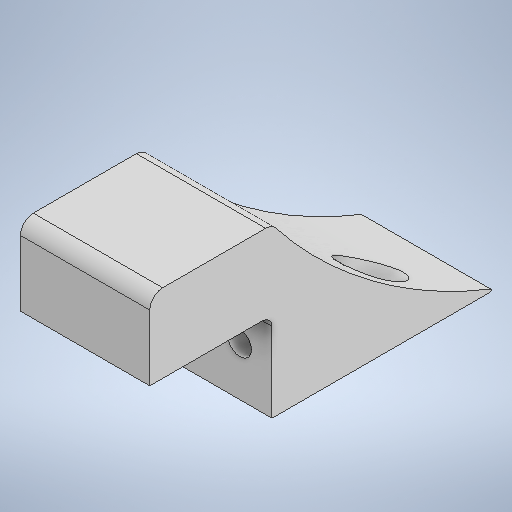
# Autodesk Inventor part: intake ramp piece
Saved by Autodesk Inventor 2025.2 (Build 292293000, 293)
## iProperties
Created: 2024-12-04
Part Number: intake ramp piece
Material: Generic
Document SubType Name: Modeling
Designer: Hunter Mathis
Density: 1 g/cm^3
Appearance: Default
Author: Hunter Mathis
## iProperties of the stored document Round intake ramp piece_3DPrint.ipt
Created: 2024-12-08
Part Number: Round intake ramp piece_3DPrint
Material: Generic
Document SubType Name: Modeling
Designer: AtuStem
Density: 1 g/cm^3
Appearance: Default
Author: AtuStem
Autodesk Inventor part; units mm, degrees
ref_plane "YZ Plane" through (0, 0, 0) normal (1, 0, 0) x (0, 1, 0)
ref_plane "XZ Plane" through (0, 0, 0) normal (0, 1, 0) x (-1, 0, 0)
ref_plane "XY Plane" through (0, 0, 0) normal (0, 0, 1) x (1, 0, 0)
sketch "Sketch24" plane through (0, 0, 0) normal (0, 0, 1) x (1, 0, 0)
  line L0 (0, 0) -> (177.8, 0)
  line L1 (177.8, 0) -> (177.8, 33.0962)
  line L2 (177.8, 33.0962) -> (0, 33.0962)
  line L3 (0, 33.0962) -> (0, 0)
  line L4 (88.9, 33.0962) -> (88.9, 0)
  line L5 (88.9, 0) -> (88.9, 7.3914)
  line L6 (88.9, 7.3914) -> (95.25, 7.3914)
  line L7 (94.488, 11.9634) -> (96.012, 11.9634)
  line L8 (97.536, 10.4394) -> (97.536, 8.9154)
  line L9 (96.012, 7.3914) -> (94.488, 7.3914)
  line L10 (92.964, 8.9154) -> (92.964, 10.4394)
  arc A0 (94.488, 11.9634) -> (92.964, 10.4394) centre (94.488, 10.4394) ccw
  arc A1 (97.536, 10.4394) -> (96.012, 11.9634) centre (96.012, 10.4394) ccw
  arc A2 (96.012, 7.3914) -> (97.536, 8.9154) centre (96.012, 8.9154) ccw
  arc A3 (92.964, 8.9154) -> (94.488, 7.3914) centre (94.488, 8.9154) ccw
  arc A4 (110.236, 10.4394) -> (108.712, 11.9634) centre (108.712, 10.4394) ccw
  arc A5 (108.712, 7.3914) -> (110.236, 8.9154) centre (108.712, 8.9154) ccw
  line L11 (108.712, 7.3914) -> (107.188, 7.3914)
  line L12 (105.664, 8.9154) -> (105.664, 10.4394)
  arc A6 (107.188, 11.9634) -> (105.664, 10.4394) centre (107.188, 10.4394) ccw
  arc A7 (105.664, 8.9154) -> (107.188, 7.3914) centre (107.188, 8.9154) ccw
  line L13 (107.188, 11.9634) -> (108.712, 11.9634)
  line L14 (110.236, 10.4394) -> (110.236, 8.9154)
  arc A8 (84.836, 10.4394) -> (83.312, 11.9634) centre (83.312, 10.4394) ccw
  arc A9 (83.312, 7.3914) -> (84.836, 8.9154) centre (83.312, 8.9154) ccw
  line L15 (83.312, 7.3914) -> (81.788, 7.3914)
  line L16 (80.264, 8.9154) -> (80.264, 10.4394)
  arc A10 (81.788, 11.9634) -> (80.264, 10.4394) centre (81.788, 10.4394) ccw
  arc A11 (80.264, 8.9154) -> (81.788, 7.3914) centre (81.788, 8.9154) ccw
  line L17 (81.788, 11.9634) -> (83.312, 11.9634)
  line L18 (84.836, 10.4394) -> (84.836, 8.9154)
  arc A12 (122.936, 10.4394) -> (121.412, 11.9634) centre (121.412, 10.4394) ccw
  arc A13 (121.412, 7.3914) -> (122.936, 8.9154) centre (121.412, 8.9154) ccw
  line L19 (121.412, 7.3914) -> (119.888, 7.3914)
  line L20 (118.364, 8.9154) -> (118.364, 10.4394)
  arc A14 (119.888, 11.9634) -> (118.364, 10.4394) centre (119.888, 10.4394) ccw
  arc A15 (118.364, 8.9154) -> (119.888, 7.3914) centre (119.888, 8.9154) ccw
  line L21 (119.888, 11.9634) -> (121.412, 11.9634)
  line L22 (122.936, 10.4394) -> (122.936, 8.9154)
  arc A16 (72.136, 10.4394) -> (70.612, 11.9634) centre (70.612, 10.4394) ccw
  arc A17 (70.612, 7.3914) -> (72.136, 8.9154) centre (70.612, 8.9154) ccw
  line L23 (70.612, 7.3914) -> (69.088, 7.3914)
  line L24 (67.564, 8.9154) -> (67.564, 10.4394)
  arc A18 (69.088, 11.9634) -> (67.564, 10.4394) centre (69.088, 10.4394) ccw
  arc A19 (67.564, 8.9154) -> (69.088, 7.3914) centre (69.088, 8.9154) ccw
  line L25 (69.088, 11.9634) -> (70.612, 11.9634)
  line L26 (72.136, 10.4394) -> (72.136, 8.9154)
  arc A20 (135.636, 10.4394) -> (134.112, 11.9634) centre (134.112, 10.4394) ccw
  arc A21 (134.112, 7.3914) -> (135.636, 8.9154) centre (134.112, 8.9154) ccw
  line L27 (134.112, 7.3914) -> (132.588, 7.3914)
  line L28 (131.064, 8.9154) -> (131.064, 10.4394)
  arc A22 (132.588, 11.9634) -> (131.064, 10.4394) centre (132.588, 10.4394) ccw
  arc A23 (131.064, 8.9154) -> (132.588, 7.3914) centre (132.588, 8.9154) ccw
  line L29 (132.588, 11.9634) -> (134.112, 11.9634)
  line L30 (135.636, 10.4394) -> (135.636, 8.9154)
  arc A24 (59.436, 10.4394) -> (57.912, 11.9634) centre (57.912, 10.4394) ccw
  arc A25 (57.912, 7.3914) -> (59.436, 8.9154) centre (57.912, 8.9154) ccw
  line L31 (57.912, 7.3914) -> (56.388, 7.3914)
  line L32 (54.864, 8.9154) -> (54.864, 10.4394)
  arc A26 (56.388, 11.9634) -> (54.864, 10.4394) centre (56.388, 10.4394) ccw
  arc A27 (54.864, 8.9154) -> (56.388, 7.3914) centre (56.388, 8.9154) ccw
  line L33 (56.388, 11.9634) -> (57.912, 11.9634)
  line L34 (59.436, 10.4394) -> (59.436, 8.9154)
  arc A28 (148.336, 10.4394) -> (146.812, 11.9634) centre (146.812, 10.4394) ccw
  arc A29 (146.812, 7.3914) -> (148.336, 8.9154) centre (146.812, 8.9154) ccw
  line L35 (146.812, 7.3914) -> (145.288, 7.3914)
  line L36 (143.764, 8.9154) -> (143.764, 10.4394)
  arc A30 (145.288, 11.9634) -> (143.764, 10.4394) centre (145.288, 10.4394) ccw
  arc A31 (143.764, 8.9154) -> (145.288, 7.3914) centre (145.288, 8.9154) ccw
  line L37 (145.288, 11.9634) -> (146.812, 11.9634)
  line L38 (148.336, 10.4394) -> (148.336, 8.9154)
  arc A32 (46.736, 10.4394) -> (45.212, 11.9634) centre (45.212, 10.4394) ccw
  arc A33 (45.212, 7.3914) -> (46.736, 8.9154) centre (45.212, 8.9154) ccw
  line L39 (45.212, 7.3914) -> (43.688, 7.3914)
  line L40 (42.164, 8.9154) -> (42.164, 10.4394)
  arc A34 (43.688, 11.9634) -> (42.164, 10.4394) centre (43.688, 10.4394) ccw
  arc A35 (42.164, 8.9154) -> (43.688, 7.3914) centre (43.688, 8.9154) ccw
  line L41 (43.688, 11.9634) -> (45.212, 11.9634)
  line L42 (46.736, 10.4394) -> (46.736, 8.9154)
  arc A36 (161.036, 10.4394) -> (159.512, 11.9634) centre (159.512, 10.4394) ccw
  arc A37 (159.512, 7.3914) -> (161.036, 8.9154) centre (159.512, 8.9154) ccw
  line L43 (159.512, 7.3914) -> (157.988, 7.3914)
  line L44 (156.464, 8.9154) -> (156.464, 10.4394)
  arc A38 (157.988, 11.9634) -> (156.464, 10.4394) centre (157.988, 10.4394) ccw
  arc A39 (156.464, 8.9154) -> (157.988, 7.3914) centre (157.988, 8.9154) ccw
  line L45 (157.988, 11.9634) -> (159.512, 11.9634)
  line L46 (161.036, 10.4394) -> (161.036, 8.9154)
  point P0 (95.25, 9.6774)
  point P1 (95.25, 7.3914)
  point P2 (107.95, 7.3914)
  point P3 (107.95, 9.6774)
  point P4 (107.95, 7.3914)
  point P5 (82.55, 7.3914)
  point P6 (82.55, 9.6774)
  point P7 (82.55, 7.3914)
  point P8 (120.65, 7.3914)
  point P9 (120.65, 9.6774)
  point P10 (120.65, 7.3914)
  point P11 (69.85, 7.3914)
  point P12 (69.85, 9.6774)
  point P13 (69.85, 7.3914)
  point P14 (133.35, 7.3914)
  point P15 (133.35, 9.6774)
  point P16 (133.35, 7.3914)
  point P17 (57.15, 7.3914)
  point P18 (57.15, 9.6774)
  point P19 (57.15, 7.3914)
  point P20 (146.05, 7.3914)
  point P21 (146.05, 9.6774)
  point P22 (146.05, 7.3914)
  point P23 (44.45, 7.3914)
  point P24 (44.45, 9.6774)
  point P25 (44.45, 7.3914)
  point P26 (158.75, 7.3914)
  point P27 (158.75, 9.6774)
  point P28 (158.75, 7.3914)
  dimension "d106" = 177.8
  dimension "d107" = 33.0962
  dimension "d119" = 7.3914
  dimension "d120" = 6.35
  dimension "d121" = 1.524
  dimension "d180" = 12.7
  constraints: 94 end point, 80 point on circle, 40 centre point, 8 tangent, 4 parallel, 3 equal radius, 3 horizontal, 3 midpoint, 3 perpendicular, 1 point on line, 207 other
  measures "d106" distance of L2.end L1.end
  measures "d107" distance of L0.end L1.end
  measures "d119" distance of L4.end L5.end
  measures "d120" distance of L5.end L6.end
  measures "d121" radius of A0
  measures "d180" distance of A1.centre A4.centre
sketch "Sketch26" plane through (0, 0, 0) normal (1, 0, 0) x (0, 1, 0)
  line L0 (0, 0) -> (0, -44.45)
  line L1 (33.0962, 0) -> (0, 0) projected
  arc A0 (33.0962, 0) -> (0, -44.45) centre (95.48, -80.9954) ccw
  dimension "d108" = 44.45
  dimension "d109" = 102.235
  constraints: 2 end point, 2 point on circle, 1 centre point, 1 vertical
  measures "d108" distance of L0.start L0.end
  measures "d109" radius of A0
extrude "Extrusion23" add sketch "Sketch26" along normal blind 177.8
sketch "Sketch27" plane through (0, 0, 0) normal (0, 0, 1) x (1, 0, 0)
  line L0 (0, 0) -> (44.45, 0)
  line L1 (0, 0) -> (177.8, 0) projected
  line L2 (44.45, 0) -> (44.45, 33.0962)
  line L3 (0, 33.0962) -> (177.8, 33.0962) projected
  arc A0 (0, 0) -> (44.45, 33.0962) centre (-36.5454, 95.48) ccw
  line L4 (0, 33.0962) -> (0, 0) projected
  line L5 (0, 0) -> (0, 33.0962)
  line L6 (0, 33.0962) -> (44.45, 33.0962)
  line L7 (0, 33.0962) -> (-19.05, 33.0962)
  line L8 (-19.05, 33.0962) -> (-19.05, 0)
  line L9 (-19.05, 0) -> (0, 0)
  line L10 (0, 0) -> (0, 33.0962)
  dimension "d112" = 44.45
  dimension "d113" = 102.235
  dimension "d114" = 19.05
  constraints: 16 end point, 3 equal length, 3 perpendicular, 2 point on circle, 2 point on line, 1 centre point, 1 horizontal
  measures "d112" distance of L0.start L0.end
  measures "d113" radius of A0
  measures "d114" distance of L9.end L8.end
revolve "Revolution1" [suppressed]
ref_plane "Work Plane3" through (88.9, 33.0962, 0) normal (-1, 0, 0) x (0, -1, 0)
mirror "Mirror1" [suppressed]
extrude "Extrusion24" add sketch "Sketch24" along normal blind 1.6002 contours A3 L10 A0 L7 A1 L8 A2 L9 L6 | L18 A9 L15 A11 L16 A10 L17 A8 | L22 A13 L19 A15 L20 A14 L21 A12 | L34 A25 L31 A27 L32 A26 L33 A24
ref_plane "Work Plane4" through (44.45, 32.1705, -50.8) normal (0, 0, 1) x (1, 0, 0)
sketch "Sketch28" plane through (44.45, 32.1705, -50.8) normal (0, 0, 1) x (1, 0, 0)
  line L0 (27.686, -23.2551) -> (27.686, -21.7311) projected
  arc A0 (27.686, -21.7311) -> (26.162, -20.2071) centre (26.162, -21.7311) ccw projected
  line L1 (26.162, -20.2071) -> (24.638, -20.2071) projected
  arc A1 (24.638, -20.2071) -> (23.114, -21.7311) centre (24.638, -21.7311) ccw projected
  line L2 (23.114, -21.7311) -> (23.114, -23.2551) projected
  arc A2 (23.114, -23.2551) -> (24.638, -24.7791) centre (24.638, -23.2551) ccw projected
  line L3 (24.638, -24.7791) -> (26.162, -24.7791) projected
  arc A3 (26.162, -24.7791) -> (27.686, -23.2551) centre (26.162, -23.2551) ccw projected
  line L4 (65.786, -23.2551) -> (65.786, -21.7311) projected
  arc A4 (65.786, -21.7311) -> (64.262, -20.2071) centre (64.262, -21.7311) ccw projected
  line L5 (64.262, -20.2071) -> (62.738, -20.2071) projected
  arc A5 (62.738, -20.2071) -> (61.214, -21.7311) centre (62.738, -21.7311) ccw projected
  line L6 (61.214, -21.7311) -> (61.214, -23.2551) projected
  arc A6 (61.214, -23.2551) -> (62.738, -24.7791) centre (62.738, -23.2551) ccw projected
  line L7 (62.738, -24.7791) -> (64.262, -24.7791) projected
  arc A7 (64.262, -24.7791) -> (65.786, -23.2551) centre (64.262, -23.2551) ccw projected
  line L8 (91.186, -23.2551) -> (91.186, -21.7311) projected
  arc A8 (91.186, -21.7311) -> (89.662, -20.2071) centre (89.662, -21.7311) ccw projected
  line L9 (89.662, -20.2071) -> (88.138, -20.2071) projected
  arc A9 (88.138, -20.2071) -> (86.614, -21.7311) centre (88.138, -21.7311) ccw projected
  line L10 (86.614, -21.7311) -> (86.614, -23.2551) projected
  arc A10 (86.614, -23.2551) -> (88.138, -24.7791) centre (88.138, -23.2551) ccw projected
  line L11 (88.138, -24.7791) -> (89.662, -24.7791) projected
  arc A11 (89.662, -24.7791) -> (91.186, -23.2551) centre (89.662, -23.2551) ccw projected
  line L12 (2.286, -23.2551) -> (2.286, -21.7311) projected
  arc A12 (2.286, -21.7311) -> (0.762, -20.2071) centre (0.762, -21.7311) ccw projected
  line L13 (0.762, -20.2071) -> (-0.762, -20.2071) projected
  arc A13 (-0.762, -20.2071) -> (-2.286, -21.7311) centre (-0.762, -21.7311) ccw projected
  line L14 (-2.286, -21.7311) -> (-2.286, -23.2551) projected
  arc A14 (-2.286, -23.2551) -> (-0.762, -24.7791) centre (-0.762, -23.2551) ccw projected
  line L15 (-0.762, -24.7791) -> (0.762, -24.7791) projected
  arc A15 (0.762, -24.7791) -> (2.286, -23.2551) centre (0.762, -23.2551) ccw projected
  line L16 (0, -32.1705) -> (0, 0.196) projected
  point P0 (-44.45, -32.1705)
sketch3d "3D Sketch1"
hole "Hole1" at (133.35, 9.6774, -25.4084) direction (0, 0, 1) diameter 4.6482 end through all start extended yes counterbore diameter 8.255 counterbore depth 5.8928
hole "Hole2" at (107.95, 9.6774, -25.4084) direction (0, 0, 1) diameter 4.6482 end through all start extended yes counterbore diameter 8.255 counterbore depth 5.8928
hole "Hole3" at (69.85, 9.6774, -25.4084) direction (0, 0, 1) diameter 4.6482 end through all start extended yes counterbore diameter 8.255 counterbore depth 5.8928
hole "Hole4" at (44.45, 9.6774, -25.4084) direction (0, 0, 1) diameter 4.6482 end through all start extended yes counterbore diameter 8.255 counterbore depth 5.8928
ref_plane "Work Plane5" through (2.0079, 0, -0.381) normal (0, -1, 0) x (1, 0, 0)
sketch "Sketch32" plane through (44.45, 0, -44.45) normal (0, -1, 0) x (1, 0, 0)
  arc A0 (-44.4489, 44.1317) -> (0, 0) centre (0, 44.45) ccw projected
  arc A1 (-44.45, 44.45) -> (0, 0) centre (0, 44.45) ccw
  arc A2 (88.9, 0) -> (133.3489, 44.1317) centre (88.9, 44.45) ccw projected
  arc A3 (88.9, 0) -> (133.3489, 44.1317) centre (88.9, 44.45) ccw
  line L0 (0, 0) -> (88.9, 0) projected
  line L1 (88.9, 0) -> (0, 0)
  arc A4 (88.9, 0) -> (133.3489, 44.1317) centre (88.9, 44.45) ccw
  arc A5 (88.9, 0) -> (133.3489, 44.1317) centre (88.9, 44.45) ccw
  line L2 (0, 0) -> (0, 12.0815) projected
  arc A6 (-44.4489, 44.1317) -> (0, 0) centre (0, 44.45) ccw
  line L3 (-43.5698, 44.45) -> (132.4698, 44.45) projected
  line L4 (132.4698, 44.45) -> (-43.5698, 44.45)
  line L5 (0, 0) -> (88.9, 0)
  arc A7 (-43.5698, 44.45) -> (-44.4489, 44.1317) centre (-43.5012, 42.8875) ccw
  arc A8 (133.3489, 44.1317) -> (132.4698, 44.45) centre (132.2102, 42.3602) ccw
  constraints: 15 point on circle, 7 centre point, 6 end point, 3 collinear
extrude "Extrusion26" [suppressed]
fillet "Fillet21" radius 0.254 1 edges at (88.9, 0, -44.45)
ref_plane "Work Plane11" through (44.45, 32.1705, 0) normal (0, 0, 1) x (1, 0, 0)
sketch "Sketch33" plane through (44.45, 32.1705, 0) normal (0, 0, 1) x (1, 0, 0)
  line L0 (-44.45, 0) -> (133.35, 0) projected
  line L1 (0, 0) -> (19.05, 0)
  line L2 (19.05, 0) -> (19.05, -33.5816)
  line L3 (0, -33.5816) -> (88.9, -33.5816) projected
  line L4 (69.7162, -33.5816) -> (69.7162, 0)
  line L5 (69.7162, 0) -> (19.05, 0)
  line L6 (19.05, 0) -> (19.05, 3.1547)
  line L7 (19.05, 3.1547) -> (69.7162, 3.1547)
  line L8 (69.7162, 3.1547) -> (69.7162, 0)
  line L9 (19.05, 0) -> (69.7162, 0)
  point P0 (-44.45, -32.1705)
  point P1 (88.9, 0)
  point P2 (69.7162, 0)
  point P3 (69.7162, 0)
  dimension "d185" = 19.05
  constraints: 16 end point, 4 perpendicular, 4 point on line, 2 equal length, 1 vertical
  measures "d185" distance of L1.start L1.end
extrude "Extrusion27" cut sketch "Sketch33" along normal through all both and the other way through all
sketch "Sketch36" plane through (44.45, -1.4111, -44.45) normal (0, -1, 0) x (1, 0, 0)
  point P0 (-44.45, 44.45)
sketch "Sketch37" plane through (177.8, 0, -43.1007) normal (0, -1, 0) x (1, 0, 0)
  line L0 (-29.7024, 55.8355) -> (18.8644, 55.8355)
  line L1 (18.8644, 55.8355) -> (18.8644, -23.5807)
  line L2 (18.8644, -23.5807) -> (-29.7024, -23.5807)
  line L3 (-29.7024, 55.8355) -> (-38.095, 55.8355)
  line L4 (-38.095, 55.8355) -> (-38.095, -23.5807)
  line L5 (-38.095, -23.5807) -> (-29.7024, -23.5807)
  point P0 (-177.8, 43.1007)
  constraints: 12 end point, 2 horizontal, 2 perpendicular, 1 collinear, 1 parallel
extrude "Extrusion28" cut sketch "Sketch37" against normal through all
ref_plane "Work Plane6" through (88.9, 0, 0) normal (1, 0, 0) x (0, 0, -1)
mirror "Mirror2" about plane through (88.9, 0, 0) normal (1, 0, 0) of "Extrusion28"
ref_plane "Work Plane12" through (114.1662, 0, 0) normal (0, 0, 1) x (1, 0, 0)
sketch "Sketch38" plane through (114.1662, 0, 0) normal (0, 0, 1) x (1, 0, 0)
  line L0 (0, 32.1642) -> (0, 20.3967)
  line L1 (0, 32.1642) -> (0, 33.0962)
  line L2 (0, 33.0962) -> (25.5009, 33.0962)
  line L3 (0, 33.0962) -> (0, 20.3967)
  line L4 (25.5388, 5.9553) -> (25.5388, 33.0962) projected
  line L5 (25.5388, 17.603) -> (0, 17.603)
  line L6 (0, 33.0962) -> (0, 0) projected
  line L7 (0, 20.3967) -> (0, 17.603)
  line L8 (-114.1662, 33.0962) -> (25.5388, 33.0962) projected
  line L9 (25.5009, 33.0962) -> (25.5388, 33.0962)
  line L10 (25.5388, 33.0962) -> (25.5388, 17.603)
  line L11 (25.5388, 0) -> (25.5388, 33.0962) projected
  line L12 (25.5388, 33.0962) -> (25.5388, 17.603)
  line L13 (25.5388, 33.0962) -> (25.5009, 33.0962)
  point P0 (-114.1662, 0)
  constraints: 20 end point, 3 collinear, 3 perpendicular, 2 point on line, 1 horizontal
extrude "Extrusion29" add sketch "Sketch38" along normal blind 24.13
ref_plane "Work Plane13" through (114.1662, 17.603, 24.13) normal (0, -1, 0) x (1, 0, 0)
sketch "Sketch39" plane through (114.1662, 17.603, 24.13) normal (0, -1, 0) x (1, 0, 0)
  line L0 (0, 0) -> (25.5388, 0) projected
  line L1 (0, 0) -> (0, -5.08)
  line L2 (0, -20.955) -> (0, 0) projected
  line L3 (0, -5.08) -> (6.477, -5.08)
  line L4 (5.715, -7.366) -> (7.239, -7.366)
  line L5 (8.763, -5.842) -> (8.763, -4.318)
  line L6 (7.239, -2.794) -> (5.715, -2.794)
  line L7 (4.191, -4.318) -> (4.191, -5.842)
  line L8 (4.191, -7.366) -> (8.763, -2.794) construction
  line L9 (8.763, -7.366) -> (4.191, -2.794) construction
  arc A0 (7.239, -7.366) -> (8.763, -5.842) centre (7.239, -5.842) ccw
  arc A1 (4.191, -5.842) -> (5.715, -7.366) centre (5.715, -5.842) ccw
  arc A2 (5.715, -2.794) -> (4.191, -4.318) centre (5.715, -4.318) ccw
  arc A3 (8.763, -4.318) -> (7.239, -2.794) centre (7.239, -4.318) ccw
  arc A4 (4.191, -18.542) -> (5.715, -20.066) centre (5.715, -18.542) ccw
  line L10 (5.715, -20.066) -> (7.239, -20.066)
  line L11 (8.763, -20.066) -> (4.191, -15.494) construction
  arc A5 (7.239, -20.066) -> (8.763, -18.542) centre (7.239, -18.542) ccw
  line L12 (8.763, -18.542) -> (8.763, -17.018)
  arc A6 (8.763, -17.018) -> (7.239, -15.494) centre (7.239, -17.018) ccw
  line L13 (7.239, -15.494) -> (5.715, -15.494)
  arc A7 (5.715, -15.494) -> (4.191, -17.018) centre (5.715, -17.018) ccw
  line L14 (0, -17.78) -> (6.477, -17.78)
  line L15 (4.191, -17.018) -> (4.191, -18.542)
  line L16 (6.477, -17.78) -> (6.477, -5.08)
  line L17 (6.477, -17.78) -> (6.477, -11.43)
  line L18 (6.477, -11.43) -> (12.827, -11.43)
  line L19 (12.065, -13.716) -> (13.589, -13.716)
  line L20 (15.113, -12.192) -> (15.113, -10.668)
  line L21 (13.589, -9.144) -> (12.065, -9.144)
  line L22 (10.541, -10.668) -> (10.541, -12.192)
  line L23 (10.541, -13.716) -> (15.113, -9.144) construction
  line L24 (15.113, -13.716) -> (10.541, -9.144) construction
  arc A8 (10.541, -12.192) -> (12.065, -13.716) centre (12.065, -12.192) ccw
  arc A9 (12.065, -9.144) -> (10.541, -10.668) centre (12.065, -10.668) ccw
  arc A10 (15.113, -10.668) -> (13.589, -9.144) centre (13.589, -10.668) ccw
  arc A11 (13.589, -13.716) -> (15.113, -12.192) centre (13.589, -12.192) ccw
  point P0 (-114.1662, -24.13)
  point P1 (4.191, -20.066)
  point P2 (8.763, -15.494)
  dimension "d198" = 5.08
  dimension "d199" = 6.477
  dimension "d201" = 4.572
  dimension "d202" = 4.572
  dimension "d203" = 1.524
  dimension "d209" = 12.7
  dimension "d214" = 6.35
  dimension "d215" = 4.572
  dimension "d216" = 4.572
  dimension "d217" = 1.524
  constraints: 46 end point, 25 point on line, 24 point on circle, 16 tangent, 12 centre point, 6 equal radius, 5 midpoint, 4 parallel, 3 horizontal, 3 perpendicular, 2 vertical, 28 other
  measures "d198" distance of L0.start L1.end
  measures "d199" distance of L1.end L3.end
  measures "d201" distance between parallel lines of L6 L4
  measures "d202" distance between parallel lines of L7 L5
  measures "d203" radius of A0
  measures "d209" distance of A1.centre A4.centre
  measures "d214" distance of L17.end L18.end
  measures "d215" distance of L23.start L24.start
  measures "d216" distance between parallel lines of L21 L19
  measures "d217" radius of A8
extrude "Extrusion30" add sketch "Sketch39" along normal blind 1.6002 contours L15 A7 L13 L16 L14 | L14 L16 L13 A6 L12 A5 L10 A4 L15 | L7 A2 L6 A3 L5 A0 L4 L16 L3 | L3 L16 L4 A1 L7 | A8 L22 A9 L21 A10 L20 A11 L19
fillet "Fillet25" radius 2.54 1 edges at (126.9356, 33.0962, 0)
sketch "Sketch40" plane through (63.5, 0, 0) normal (0, 0, 1) x (1, 0, 0)
  line L0 (8.2246, 40.0148) -> (-39.0885, 40.0148)
  line L1 (-39.0885, 40.0148) -> (-39.0885, -10.9894)
  line L2 (-39.0885, -10.9894) -> (8.2246, -10.9894)
  line L3 (8.2246, -10.9894) -> (8.2246, 40.0148)
  point P0 (-63.5, 0)
  constraints: 8 end point, 2 parallel, 1 horizontal, 1 perpendicular
extrude "Extrusion31" cut sketch "Sketch40" along normal through all both and the other way through all
fillet "Fillet26" radius 1.905 1 edges at (126.9356, 17.603, 0)
fillet "Fillet27" radius 2.54 1 edges at (126.9356, 33.0962, 24.13)
body "Solid2"
